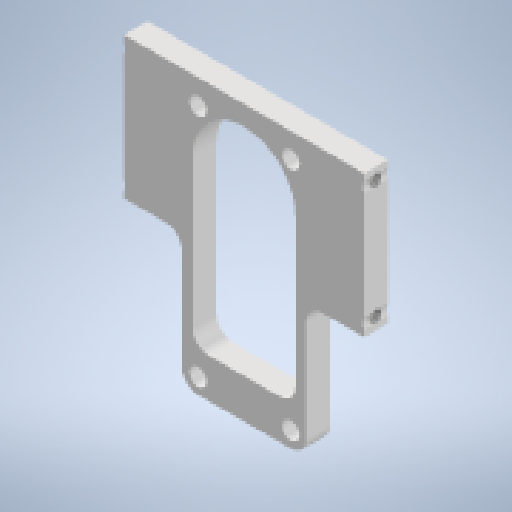
# Autodesk Inventor part: udeyo
Saved by Autodesk Inventor 2024 (Build 280153000, 153)
## iProperties
Created: 2023-12-31
Part Number: udeyo
Material: 一般
Document SubType Name: Modeling
Designer: right
Density: 1 g/cm^3
Appearance: 既定
Author: right
Autodesk Inventor part; units mm, degrees
ref_plane "YZ Plane" through (0, 0, 0) normal (1, 0, 0) x (0, 1, 0)
ref_plane "XZ Plane" through (0, 0, 0) normal (0, 1, 0) x (-1, 0, 0)
ref_plane "XY Plane" through (0, 0, 0) normal (0, 0, 1) x (1, 0, 0)
sketch "スケッチ1" plane through (0, 0, 0) normal (0, 0, 1) x (1, 0, 0)
  line L0 (-5.9, -14.9) -> (5.9, -14.9) construction
  line L1 (5.9, -14.9) -> (5.9, 14.9) construction
  line L2 (5.9, 14.9) -> (-5.9, 14.9) construction
  line L3 (-5.9, 14.9) -> (-5.9, -14.9) construction
  line L4 (-5.9, -14.9) -> (5.9, 14.9) construction
  line L5 (5.9, -14.9) -> (-5.9, 14.9) construction
  circle A0 centre (-5.9, 14.9) radius 1.1
  circle A1 centre (-5.9, 14.9) radius 2
  circle A2 centre (5.9, 14.9) radius 2
  circle A3 centre (5.9, 14.9) radius 1.1
  circle A4 centre (-5.9, -14.9) radius 2
  circle A5 centre (-5.9, -14.9) radius 1.1
  circle A6 centre (5.9, -14.9) radius 2
  circle A7 centre (5.9, -14.9) radius 1.1
  circle A8 centre (0, 8.9998) radius 6.5
  circle A9 centre (-5.9, 14.9) radius 8.344 construction
  line L6 (-6.5, 8.9998) -> (6.5, 8.9998)
  line L7 (6.5, 8.9998) -> (6.5, -11.9)
  line L8 (6.5, -11.9) -> (-6.5, -11.9)
  line L9 (-6.5, -11.9) -> (-6.5, 8.9998)
  line L10 (-7.9, -16.9) -> (7.9, -16.9)
  line L11 (7.9, -16.9) -> (7.9, 16.9)
  line L12 (7.9, 16.9) -> (-7.9, 16.9)
  line L13 (-7.9, 16.9) -> (-7.9, -16.9)
  line L14 (-7.9, -16.9) -> (7.9, 16.9) construction
  line L15 (7.9, -16.9) -> (-7.9, 16.9) construction
  line L16 (-15.25, -0.0002) -> (15.25, -0.0002)
  line L17 (15.25, -0.0002) -> (15.25, 17.9998)
  line L18 (15.25, 17.9998) -> (-15.25, 17.9998)
  line L19 (-15.25, 17.9998) -> (-15.25, -0.0002)
  line L20 (-15.25, -0.0002) -> (15.25, 17.9998) construction
  line L21 (15.25, -0.0002) -> (-15.25, 17.9998) construction
  point P0 (0, 0)
  point P1 (0, 14.9)
  point P2 (7.9, -0.0002)
  point P3 (-7.9, -0.0002)
  point P4 (-7.9, -14.9)
  point P5 (-5.9, -16.9)
  point P6 (5.9, -16.9)
  point P7 (7.9, -14.9)
  point P8 (6.5, 8.9998)
  dimension "d12" = 13
  dimension "d13" = 16.688
  dimension "d0" = 11.8
  dimension "d1" = 29.8
  dimension "d2" = 2.2
  dimension "d3" = 4
  dimension "d6" = 11.8
  dimension "d9" = 29.8
  dimension "d14" = 3
  dimension "d15" = 30.5
  dimension "d16" = 18
  constraints: 44 end point, 8 centre point, 8 parallel, 7 midpoint, 6 coincident, 5 horizontal, 4 perpendicular, 3 vertical, 2 tangent, 1 vertical alignment, 18 other
  measures "d0" distance of L1.end L2.end
  measures "d1" distance of L2.end L0.start
  measures "d2" diameter of A0
  measures "d3" diameter of A1
  measures "d6" distance of A1.centre A2.centre
  measures "d9" distance of A1.centre A4.centre
  measures "d14" distance from line of L8 A6.centre
  measures "d15" distance of L18.end L17.end
  measures "d16" distance of L18.end L16.start
extrude "押し出し1" add sketch "スケッチ1" along normal blind 3 contours A1 A8 | A1 L12 A2 A8 | L12 L13 L16 L19 L18 L17 L11 | A1 L13 L12 | A1 A8 L9 L16 L13 | L12 L11 A2 | A2 A8 | L16 L9 L8 L7 L11 A6 L10 A4 L13 | L11 L16 L7 A8 A2 | A4 | A6 picked at (-7.5833, 15.0483) picked at (7.5833, 15.0483)
fillet "フィレット1" radius 2 4 edges at (-7.9, -0.0002, 1.5) (7.9, -0.0002, 1.5) (-6.5, -11.9, 1.5) (6.5, -11.9, 1.5)
sketch "スケッチ2" plane through (-15.25, -0.0002, 0) normal (-1, 0, 0) x (0, 0, 1)
  line L0 (0, 18) -> (3, 18) construction
  line L1 (1.5, 18) -> (1.5, 0) construction
  line L2 (0, 0) -> (3, 0) construction
  line L3 (0, 9) -> (3, 9) construction
  line L4 (1.5, 9) -> (3, 9) construction
  point P0 (0, 0.0002)
  point P1 (1.5, 16.5)
  point P2 (1.5, 1.5)
  dimension "d20" = 15
  constraints: 4 end point, 3 midpoint, 1 horizontal, 1 point on line, 1 symmetric about line
  measures "d20" distance of point (1.5, 1.5) point (1.5, 16.5)
hole "穴1" at (-15.25, 16.4998, 1.5) at (-15.25, 1.4998, 1.5) direction (1, 0, 0) diameter 1.567 depth 4.5 tip angle 118 thread size "M2x0.4" class "6H" standard "ISO Metric profile"
sketch "スケッチ3" plane through (15.25, -0.0002, 0) normal (1, 0, 0) x (0, 0, -1)
  line L0 (0, 0) -> (0, 18) projected
  circle A0 centre (-1.5, 1.5) radius 0.7835 projected
  circle A1 centre (-1.5, 16.5) radius 0.7835 projected
  line L1 (0, 18) -> (0, 0) projected
  line L2 (0, 0) -> (-3, 0) projected
  line L3 (-3, 18) -> (-3, 0) projected
  line L4 (0, 18) -> (-3, 18) projected
  point P0 (0, 0.0002)
  constraints: 2 coincident
hole "穴2" at (15.25, 1.4998, 1.5) at (15.25, 16.4998, 1.5) direction (-1, 0, 0) diameter 1.567 depth 4.5 tip angle 118 thread size "M2x0.4" class "6H" standard "ISO Metric profile"
sketch "スケッチ4" plane through (0, 0, 3) normal (0, 0, 1) x (1, 0, 0)
  line L0 (-15.25, 0.7163) -> (-15.25, 2.2833) projected
  line L1 (-15.25, 15.7163) -> (-15.25, 17.2833) projected
  circle A0 centre (-16.15, 1.4998) radius 1.1
  line L2 (-15.25, 17.9998) -> (-15.25, -0.0002) construction
  line L3 (-15.25, 8.9998) -> (15.25, 8.9998) construction
  line L4 (15.25, -0.0002) -> (15.25, 17.9998) construction
  line L5 (15.25, 17.9998) -> (-15.25, 17.9998) construction
  line L6 (0, 17.9998) -> (0, 8.9998) construction
  circle A1 centre (-16.15, 16.4998) radius 1.1
  line L7 (15.25, 0.7163) -> (15.25, 2.2833)
  line L8 (15.25, 15.7163) -> (15.25, 17.2833)
  circle A2 centre (16.15, 1.4998) radius 1.1
  line L9 (15.25, 17.9998) -> (15.25, -0.0002) construction
  circle A3 centre (16.15, 16.4998) radius 1.1
  point P0 (0, 0)
  point P1 (-15.25, 1.4998)
  point P2 (15.25, 1.4998)
  dimension "d35" = 2.2
  dimension "d36" = 0.9
  constraints: 10 end point, 8 symmetric about line, 5 midpoint, 4 centre point, 1 horizontal alignment, 3 other
  measures "d35" diameter of A0
  measures "d36" distance from line of L0 A0.centre
extrude "押し出し2" cut sketch "スケッチ4" against normal blind 3
equation "\"d6\" = d0"
equation "\"d9\" = d1"
